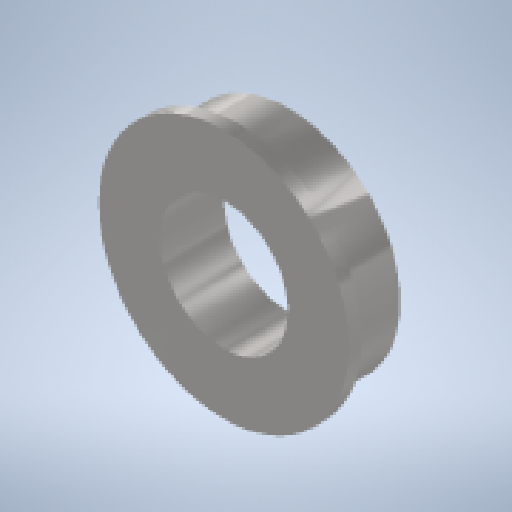
# Autodesk Inventor part: SMF148ZZ
Saved by Autodesk Inventor 2024 (Build 280153000, 153)
## iProperties
Created: 2023-05-26
Part Number: SMF148ZZ
Material: 鋼、炭素鋼
Document SubType Name: Modeling
Designer: yuta2
Density: 7.85 g/cm^3
Appearance: 半つや出し
Author: yuta2
Autodesk Inventor part; units mm, degrees
ref_plane "YZ Plane" through (0, 0, 0) normal (1, 0, 0) x (0, 1, 0)
ref_plane "XZ Plane" through (0, 0, 0) normal (0, 1, 0) x (-1, 0, 0)
ref_plane "XY Plane" through (0, 0, 0) normal (0, 0, 1) x (1, 0, 0)
sketch "スケッチ1" plane through (0, 0, 0) normal (1, 0, 0) x (0, 1, 0)
  line L0 (0, 0) -> (4, 0)
  line L1 (4, 0) -> (4, -4)
  line L2 (4, -4) -> (0, -4)
  line L3 (0, -4) -> (0, 0)
  line L4 (0, 0) -> (7, 0)
  line L5 (7, 0) -> (7, -4)
  line L6 (7, -4) -> (0, -4)
  line L7 (0, -4) -> (0, 0)
  line L8 (7, 0) -> (7.8, 0)
  line L9 (7.8, 0) -> (7.8, -0.8)
  line L10 (7.8, -0.8) -> (7, -0.8)
  line L11 (7, -0.8) -> (7, 0)
  dimension "d0" = 4
  dimension "d1" = 4
  dimension "d2" = 7
  dimension "d3" = 0.8
  dimension "d4" = 0.8
  constraints: 24 end point, 6 parallel, 3 horizontal, 3 perpendicular, 1 collinear
  measures "d0" distance of L1.end L2.end
  measures "d1" distance of L0.end L1.end
  measures "d2" distance of L5.end L6.end
  measures "d3" distance of L9.end L10.end
  measures "d4" distance of L8.end L9.end
revolve "回転1" add sketch "スケッチ1" angle 360 about axis through (0, 0, -4) along (0, 0, 1) contours L4 L5 L6 L1 | L8 L9 L10 L5
